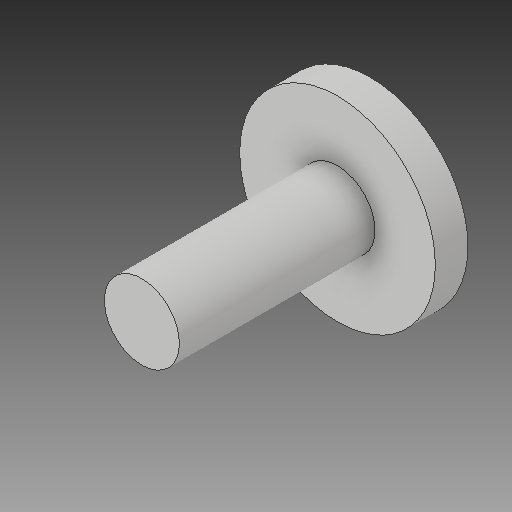
# Autodesk Inventor part: Frame mount rivet
Saved by Autodesk Inventor 2018 (Build 220112000, 112)
## iProperties
Created: 2018-03-18
Part Number: Frame mount rivet
Material: Generic
Document SubType Name: Modeling
Designer: MIABo
Density: 1 g/cm^3
Appearance: Default
Mass: 0.871839 g
Surface Area: 7.66142 cm^2
Volume: 0.871839 cm^3
Author: MIABo
## iProperties of the stored document Frame mount rivet_3DPrint.ipt
Created: 2018-03-20
Part Number: Frame mount rivet_3DPrint
Material: Generic
Document SubType Name: Modeling
Designer: MIABo
Density: 1 g/cm^3
Appearance: Default
Author: MIABo
Autodesk Inventor part; units mm, degrees
ref_plane "YZ Plane" through (0, 0, 0) normal (1, 0, 0) x (0, 1, 0)
ref_plane "XZ Plane" through (0, 0, 0) normal (0, 1, 0) x (-1, 0, 0)
ref_plane "XY Plane" through (0, 0, 0) normal (0, 0, 1) x (1, 0, 0)
sketch "Sketch1" plane through (0, 0, 0) normal (0, 0, 1) x (1, 0, 0)
  circle A0 centre (0, 0) radius 7.62
  dimension "d0" = 15.24
  constraints: 1 centre point, 1 coincident
  measures "d0" diameter of A0
extrude "Extrusion1" add sketch "Sketch1" along normal blind 2.54
sketch "Sketch2" plane through (0, 0, 2.54) normal (0, 0, 1) x (1, 0, 0)
  circle A0 centre (0, 0) radius 2.921
  dimension "d3" = 5.842
  constraints: 1 centre point, 1 coincident
  measures "d3" diameter of A0
extrude "Extrusion2" add sketch "Sketch2" along normal blind 15.24
body "Solid1"
